Autodesk Fusion 360 part; units mm, degrees
note: some values were not read from the file. Set by a fixed rule: which sketch regions a step uses.
(part 3 of 20)
  spline S12 degree 5 poles (15.9204, -26.5997) (15.9199, -26.597) (15.9189, -26.5917) (15.9174, -26.5837) (15.9154, -26.5731) (15.913, -26.5599) (15.9105, -26.5467) (15.908, -26.5335) (15.9055, -26.5204) (15.9029, -26.5073) (15.9004, -26.4943) (15.8979, -26.4812) (15.8953, -26.4682) (15.8927, -26.4553) (15.8902, -26.4424) (15.8876, -26.4295) (15.885, -26.4166) (15.8824, -26.4038) (15.8798, -26.391) (15.8771, -26.3783) (15.8745, -26.3656) (15.8719, -26.3529) (15.8692, -26.3403) (15.8666, -26.3276) (15.8639, -26.3151) (15.8612, -26.3025) (15.8585, -26.29) (15.8558, -26.2776) (15.8531, -26.2651) (15.8504, -26.2528) (15.8477, -26.2404) (15.8449, -26.2281) (15.8422, -26.2158) (15.8394, -26.2035) (15.8367, -26.1913) (15.8339, -26.1792) (15.8311, -26.167) (15.8283, -26.1549) (15.8255, -26.1428) (15.8227, -26.1308) (15.8199, -26.1188) (15.8171, -26.1069) (15.8143, -26.095) (15.8115, -26.0831) (15.8086, -26.0712) (15.8058, -26.0594) (15.8029, -26.0477) (15.8001, -26.0359) (15.7972, -26.0242) (15.7943, -26.0126) (15.7914, -26.001) (15.7886, -25.9894) (15.7857, -25.9778) (15.7828, -25.9663) (15.7798, -25.9549) (15.7769, -25.9435) (15.774, -25.9321) (15.7711, -25.9207) (15.7682, -25.9094) (15.7652, -25.8982) (15.7623, -25.8869) (15.7593, -25.8757) (15.7564, -25.8646) (15.7534, -25.8535) (15.7504, -25.8424) (15.7475, -25.8314) (15.7445, -25.8204) (15.7415, -25.8094) (15.7385, -25.7985) (15.7355, -25.7877) (15.7325, -25.7768) (15.7295, -25.766) (15.7265, -25.7553) (15.7235, -25.7446) (15.7205, -25.7339) (15.7175, -25.7233) (15.7145, -25.7127) (15.7114, -25.7022) (15.7084, -25.6917) (15.7054, -25.6812) (15.7023, -25.6708) (15.6993, -25.6604) (15.6963, -25.6501) (15.6932, -25.6398) (15.6902, -25.6296) (15.6871, -25.6194) (15.6841, -25.6092) (15.681, -25.5991) (15.6779, -25.589) (15.6749, -25.579) (15.6718, -25.569) (15.6688, -25.559) (15.6657, -25.5491) (15.6626, -25.5393) (15.6596, -25.5294) (15.6565, -25.5197) (15.6534, -25.5099) (15.6503, -25.5003) (15.6473, -25.4906) (15.6442, -25.481) (15.6411, -25.4715) (15.638, -25.462) (15.635, -25.4525) (15.6319, -25.4431) (15.6288, -25.4337) (15.6257, -25.4244) (15.6227, -25.4151) (15.6196, -25.4059) (15.6165, -25.3967) (15.6134, -25.3876) (15.6104, -25.3785) (15.6073, -25.3694) (15.6042, -25.3604) (15.6012, -25.3515) (15.5981, -25.3426) (15.595, -25.3337) (15.592, -25.3249) (15.5889, -25.3161) (15.5859, -25.3074) (15.5828, -25.2988) (15.5798, -25.2901) (15.5767, -25.2816) (15.5737, -25.2731) (15.5706, -25.2646) (15.5676, -25.2562) (15.5645, -25.2478) (15.5615, -25.2394) (15.5585, -25.2312) (15.5555, -25.2229) (15.5524, -25.2148) (15.5494, -25.2066) (15.5464, -25.1986) (15.5434, -25.1905) (15.5404, -25.1826) (15.5374, -25.1746) (15.5344, -25.1668) (15.5315, -25.1589) (15.5285, -25.1512) (15.5255, -25.1434) (15.5226, -25.1358) (15.5196, -25.1282) (15.5166, -25.1206) (15.5137, -25.1131) (15.5108, -25.1056) (15.5078, -25.0982) (15.5049, -25.0909) (15.502, -25.0836) (15.4991, -25.0763) (15.4962, -25.0691) (15.4933, -25.062) (15.4905, -25.0549) (15.4876, -25.0479) (15.4848, -25.0409) (15.4819, -25.034) (15.4791, -25.0271) (15.4762, -25.0203) (15.4734, -25.0136) (15.4706, -25.0069) (15.4678, -25.0002) (15.4651, -24.9936) (15.4623, -24.9871) (15.4595, -24.9806) (15.4568, -24.9742) (15.4541, -24.9679) (15.4514, -24.9616) (15.4486, -24.9553) (15.446, -24.9492) (15.4433, -24.943) (15.4406, -24.937) (15.438, -24.931) (15.4353, -24.925) (15.4327, -24.9192) (15.4301, -24.9133) (15.4275, -24.9076) (15.425, -24.9019) (15.4224, -24.8962) (15.4199, -24.8907) (15.4174, -24.8852) (15.4149, -24.8797) (15.4124, -24.8743) (15.4099, -24.869) (15.4075, -24.8637) (15.405, -24.8585) (15.4026, -24.8534) (15.4002, -24.8483) (15.3979, -24.8433) (15.3955, -24.8384) (15.3932, -24.8335) (15.3909, -24.8287) (15.3886, -24.8239) (15.3863, -24.8193) (15.3841, -24.8147) (15.3819, -24.8101) (15.3797, -24.8056) (15.3775, -24.8012) (15.3754, -24.7969) (15.3733, -24.7926) (15.3712, -24.7884) (15.3691, -24.7843) (15.3671, -24.7802) (15.3651, -24.7763) (15.3631, -24.7723) (15.3611, -24.7685) (15.3592, -24.7647) (15.3573, -24.761) (15.3554, -24.7574) (15.3536, -24.7539) (15.3518, -24.7504) (15.35, -24.747) (15.3482, -24.7437) (15.3465, -24.7404) (15.3449, -24.7372) (15.3432, -24.7341) (15.3416, -24.7311) (15.34, -24.7282) (15.3385, -24.7253) (15.337, -24.7225) (15.3355, -24.7198) (15.3341, -24.7172) (15.3327, -24.7147) (15.3313, -24.7122) (15.33, -24.7099) (15.3287, -24.7076) (15.3275, -24.7054) (15.3263, -24.7033) (15.3252, -24.7012) (15.3241, -24.6993) (15.323, -24.6974) (15.322, -24.6956) (15.321, -24.694) (15.3201, -24.6924) (15.3193, -24.6909) (15.3184, -24.6895) (15.3177, -24.6881) (15.3169, -24.6869) (15.3163, -24.6858) (15.3157, -24.6848) (15.3151, -24.6838) (15.3146, -24.683) (15.3142, -24.6822) (15.3138, -24.6816) (15.3135, -24.6812) (15.3133, -24.6809) (15.3132, -24.6807) (15.3132, -24.6806) knots -1 -1 -1 -1 -1 -1 -0.99583333 -0.99166667 -0.9875 -0.98333333 -0.97916667 -0.975 -0.97083333 -0.96666667 -0.9625 -0.95833333 -0.95416667 -0.95 -0.94583333 -0.94166667 -0.9375 -0.93333333 -0.92916667 -0.925 -0.92083333 -0.91666667 -0.9125 -0.90833333 -0.90416667 -0.9 -0.89583333 -0.89166667 -0.8875 -0.88333333 -0.87916667 -0.875 -0.87083333 -0.86666667 -0.8625 -0.85833333 -0.85416667 -0.85 -0.84583333 -0.84166667 -0.8375 -0.83333333 -0.82916667 -0.825 -0.82083333 -0.81666667 -0.8125 -0.80833333 -0.80416667 -0.8 -0.79583333 -0.79166667 -0.7875 -0.78333333 -0.77916667 -0.775 -0.77083333 -0.76666667 -0.7625 -0.75833333 -0.75416667 -0.75 -0.74583333 -0.74166667 -0.7375 -0.73333333 -0.72916667 -0.725 -0.72083333 -0.71666667 -0.7125 -0.70833333 -0.70416667 -0.7 -0.69583333 -0.69166667 -0.6875 -0.68333333 -0.67916667 -0.675 -0.67083333 -0.66666667 -0.6625 -0.65833333 -0.65416667 -0.65 -0.64583333 -0.64166667 -0.6375 -0.63333333 -0.62916667 -0.625 -0.62083333 -0.61666667 -0.6125 -0.60833333 -0.60416667 -0.6 -0.59583333 -0.59166667 -0.5875 -0.58333333 -0.57916667 -0.575 -0.57083333 -0.56666667 -0.5625 -0.55833333 -0.55416667 -0.55 -0.54583333 -0.54166667 -0.5375 -0.53333333 -0.52916667 -0.525 -0.52083333 -0.51666667 -0.5125 -0.50833333 -0.50416667 -0.5 -0.49583333 -0.49166667 -0.4875 -0.48333333 -0.47916667 -0.475 -0.47083333 -0.46666667 -0.4625 -0.45833333 -0.45416667 -0.45 -0.44583333 -0.44166667 -0.4375 -0.43333333 -0.42916667 -0.425 -0.42083333 -0.41666667 -0.4125 -0.40833333 -0.40416667 -0.4 -0.39583333 -0.39166667 -0.3875 -0.38333333 -0.37916667 -0.375 -0.37083333 -0.36666667 -0.3625 -0.35833333 -0.35416667 -0.35 -0.34583333 -0.34166667 -0.3375 -0.33333333 -0.32916667 -0.325 -0.32083333 -0.31666667 -0.3125 -0.30833333 -0.30416667 -0.3 -0.29583333 -0.29166667 -0.2875 -0.28333333 -0.27916667 -0.275 -0.27083333 -0.26666667 -0.2625 -0.25833333 -0.25416667 -0.25 -0.24583333 -0.24166667 -0.2375 -0.23333333 -0.22916667 -0.225 -0.22083333 -0.21666667 -0.2125 -0.20833333 -0.20416667 -0.2 -0.19583333 -0.19166667 -0.1875 -0.18333333 -0.17916667 -0.175 -0.17083333 -0.16666667 -0.1625 -0.15833333 -0.15416667 -0.15 -0.14583333 -0.14166667 -0.1375 -0.13333333 -0.12916667 -0.125 -0.12083333 -0.11666667 -0.1125 -0.10833333 -0.10416667 -0.1 -0.09583333 -0.09166667 -0.0875 -0.08333333 -0.07916667 -0.075 -0.07083333 -0.06666667 -0.0625 -0.05833333 -0.05416667 -0.05 -0.04583333 -0.04166667 -0.0375 -0.03333333 -0.02916667 -0.025 -0.02083333 -0.01666667 -0.0125 -0.00833333 -0.00416667 0 0 0 0 0 0
  line L22 (18.7401, 22.1898) -> (18.5501, 21.9649)
  line L23 (9.8472, -27.3251) -> (9.8469, -27.3243)
  arc A11 (15.1575, -24.4297) -> (16.1526, -23.7836) centre (0, 0) ccw
  arc A12 (15.0758, -27.0873) -> (15.9204, -26.5997) centre (0, 0) ccw
  line L24 (16.318, -24.0271) -> (16.3184, -24.0278)
  line L25 (16.1526, -23.7836) -> (16.318, -24.0271)
  line L26 (17.8086, 22.9441) -> (17.8091, 22.9448)
  spline S13 degree 5 poles (24.0278, 16.3184) (24.0279, 16.3185) (24.0281, 16.3186) (24.0283, 16.3188) (24.0287, 16.3191) (24.0294, 16.3195) (24.0301, 16.32) (24.0309, 16.3206) (24.0317, 16.3212) (24.0327, 16.3219) (24.0338, 16.3227) (24.035, 16.3235) (24.0362, 16.3244) (24.0375, 16.3253) (24.0389, 16.3263) (24.0404, 16.3274) (24.042, 16.3286) (24.0436, 16.3298) (24.0453, 16.331) (24.0471, 16.3324) (24.049, 16.3338) (24.051, 16.3352) (24.053, 16.3367) (24.0551, 16.3383) (24.0572, 16.3399) (24.0595, 16.3416) (24.0618, 16.3434) (24.0641, 16.3452) (24.0666, 16.3471) (24.0691, 16.349) (24.0717, 16.351) (24.0743, 16.353) (24.077, 16.3551) (24.0798, 16.3573) (24.0826, 16.3595) (24.0855, 16.3618) (24.0884, 16.3641) (24.0914, 16.3665) (24.0945, 16.3689) (24.0976, 16.3714) (24.1008, 16.374) (24.104, 16.3766) (24.1073, 16.3792) (24.1107, 16.3819) (24.1141, 16.3847) (24.1176, 16.3875) (24.1211, 16.3904) (24.1246, 16.3933) (24.1283, 16.3963) (24.1319, 16.3994) (24.1356, 16.4024) (24.1394, 16.4056) (24.1432, 16.4088) (24.1471, 16.412) (24.151, 16.4153) (24.155, 16.4187) (24.159, 16.4221) (24.1631, 16.4256) (24.1672, 16.4291) (24.1713, 16.4326) (24.1755, 16.4362) (24.1798, 16.4399) (24.1841, 16.4436) (24.1884, 16.4474) (24.1928, 16.4512) (24.1972, 16.455) (24.2017, 16.459) (24.2062, 16.4629) (24.2107, 16.4669) (24.2153, 16.471) (24.2199, 16.4751) (24.2246, 16.4793) (24.2293, 16.4835) (24.234, 16.4877) (24.2388, 16.492) (24.2436, 16.4964) (24.2485, 16.5008) (24.2534, 16.5053) (24.2583, 16.5098) (24.2633, 16.5143) (24.2683, 16.5189) (24.2733, 16.5236) (24.2784, 16.5282) (24.2835, 16.533) (24.2887, 16.5378) (24.2939, 16.5426) (24.2991, 16.5475) (24.3043, 16.5524) (24.3096, 16.5574) (24.3149, 16.5624) (24.3203, 16.5675) (24.3257, 16.5726) (24.3311, 16.5778) (24.3365, 16.583) (24.342, 16.5882) (24.3475, 16.5935) (24.353, 16.5989) (24.3586, 16.6043) (24.3642, 16.6097) (24.3698, 16.6152) (24.3755, 16.6207) (24.3812, 16.6263) (24.3869, 16.6319) (24.3926, 16.6376) (24.3984, 16.6433) (24.4042, 16.6491) (24.41, 16.6549) (24.4159, 16.6607) (24.4218, 16.6666) (24.4277, 16.6725) (24.4336, 16.6785) (24.4395, 16.6845) (24.4455, 16.6906) (24.4515, 16.6967) (24.4576, 16.7029) (24.4636, 16.7091) (24.4697, 16.7153) (24.4758, 16.7216) (24.482, 16.7279) (24.4881, 16.7343) (24.4943, 16.7407) (24.5005, 16.7472) (24.5067, 16.7537) (24.513, 16.7602) (24.5192, 16.7668) (24.5255, 16.7735) (24.5319, 16.7801) (24.5382, 16.7869) (24.5446, 16.7936) (24.5509, 16.8004) (24.5573, 16.8073) (24.5638, 16.8142) (24.5702, 16.8211) (24.5767, 16.8281) (24.5831, 16.8351) (24.5897, 16.8421) (24.5962, 16.8492) (24.6027, 16.8564) (24.6093, 16.8636) (24.6159, 16.8708) (24.6225, 16.8781) (24.6291, 16.8854) (24.6357, 16.8927) (24.6424, 16.9001) (24.6491, 16.9075) (24.6558, 16.915) (24.6625, 16.9225) (24.6692, 16.9301) (24.6759, 16.9377) (24.6827, 16.9453) (24.6895, 16.953) (24.6963, 16.9607) (24.7031, 16.9685) (24.7099, 16.9763) (24.7168, 16.9841) (24.7236, 16.992) (24.7305, 16.9999) (24.7374, 17.0079) (24.7443, 17.0159) (24.7512, 17.0239) (24.7582, 17.032) (24.7651, 17.0401) (24.7721, 17.0483) (24.7791, 17.0565) (24.7861, 17.0647) (24.7931, 17.073) (24.8001, 17.0813) (24.8071, 17.0897) (24.8142, 17.0981) (24.8212, 17.1065) (24.8283, 17.115) (24.8354, 17.1235) (24.8425, 17.1321) (24.8496, 17.1407) (24.8568, 17.1493) (24.8639, 17.158) (24.8711, 17.1667) (24.8782, 17.1754) (24.8854, 17.1842) (24.8926, 17.1931) (24.8998, 17.2019) (24.907, 17.2108) (24.9142, 17.2198) (24.9215, 17.2288) (24.9287, 17.2378) (24.936, 17.2469) (24.9432, 17.2559) (24.9505, 17.2651) (24.9578, 17.2743) (24.9651, 17.2835) (24.9724, 17.2927) (24.9797, 17.302) (24.9871, 17.3113) (24.9944, 17.3207) (25.0017, 17.3301) (25.0091, 17.3395) (25.0165, 17.349) (25.0238, 17.3585) (25.0312, 17.3681) (25.0386, 17.3777) (25.046, 17.3873) (25.0534, 17.397) (25.0609, 17.4067) (25.0683, 17.4164) (25.0757, 17.4262) (25.0832, 17.436) (25.0906, 17.4458) (25.0981, 17.4557) (25.1055, 17.4657) (25.113, 17.4756) (25.1205, 17.4856) (25.128, 17.4956) (25.1355, 17.5057) (25.143, 17.5158) (25.1505, 17.526) (25.158, 17.5361) (25.1655, 17.5464) (25.1731, 17.5566) (25.1806, 17.5669) (25.1881, 17.5772) (25.1957, 17.5876) (25.2032, 17.598) (25.2108, 17.6084) (25.2184, 17.6189) (25.2259, 17.6294) (25.2335, 17.6399) (25.2411, 17.6505) (25.2487, 17.6611) (25.2563, 17.6718) (25.2639, 17.6825) (25.2715, 17.6932) (25.2791, 17.7039) (25.2867, 17.7147) (25.2943, 17.7256) (25.3019, 17.7364) (25.3096, 17.7473) (25.3172, 17.7583) (25.3248, 17.7692) (25.3325, 17.7802) (25.3401, 17.7913) (25.3477, 17.8023) (25.3539, 17.8112) (25.3584, 17.8179) (25.3615, 17.8224) (25.363, 17.8246) knots 0 0 0 0 0 0 0.00416667 0.00833333 0.0125 0.01666667 0.02083333 0.025 0.02916667 0.03333333 0.0375 0.04166667 0.04583333 0.05 0.05416667 0.05833333 0.0625 0.06666667 0.07083333 0.075 0.07916667 0.08333333 0.0875 0.09166667 0.09583333 0.1 0.10416667 0.10833333 0.1125 0.11666667 0.12083333 0.125 0.12916667 0.13333333 0.1375 0.14166667 0.14583333 0.15 0.15416667 0.15833333 0.1625 0.16666667 0.17083333 0.175 0.17916667 0.18333333 0.1875 0.19166667 0.19583333 0.2 0.20416667 0.20833333 0.2125 0.21666667 0.22083333 0.225 0.22916667 0.23333333 0.2375 0.24166667 0.24583333 0.25 0.25416667 0.25833333 0.2625 0.26666667 0.27083333 0.275 0.27916667 0.28333333 0.2875 0.29166667 0.29583333 0.3 0.30416667 0.30833333 0.3125 0.31666667 0.32083333 0.325 0.32916667 0.33333333 0.3375 0.34166667 0.34583333 0.35 0.35416667 0.35833333 0.3625 0.36666667 0.37083333 0.375 0.37916667 0.38333333 0.3875 0.39166667 0.39583333 0.4 0.40416667 0.40833333 0.4125 0.41666667 0.42083333 0.425 0.42916667 0.43333333 0.4375 0.44166667 0.44583333 0.45 0.45416667 0.45833333 0.4625 0.46666667 0.47083333 0.475 0.47916667 0.48333333 0.4875 0.49166667 0.49583333 0.5 0.50416667 0.50833333 0.5125 0.51666667 0.52083333 0.525 0.52916667 0.53333333 0.5375 0.54166667 0.54583333 0.55 0.55416667 0.55833333 0.5625 0.56666667 0.57083333 0.575 0.57916667 0.58333333 0.5875 0.59166667 0.59583333 0.6 0.60416667 0.60833333 0.6125 0.61666667 0.62083333 0.625 0.62916667 0.63333333 0.6375 0.64166667 0.64583333 0.65 0.65416667 0.65833333 0.6625 0.66666667 0.67083333 0.675 0.67916667 0.68333333 0.6875 0.69166667 0.69583333 0.7 0.70416667 0.70833333 0.7125 0.71666667 0.72083333 0.725 0.72916667 0.73333333 0.7375 0.74166667 0.74583333 0.75 0.75416667 0.75833333 0.7625 0.76666667 0.77083333 0.775 0.77916667 0.78333333 0.7875 0.79166667 0.79583333 0.8 0.80416667 0.80833333 0.8125 0.81666667 0.82083333 0.825 0.82916667 0.83333333 0.8375 0.84166667 0.84583333 0.85 0.85416667 0.85833333 0.8625 0.86666667 0.87083333 0.875 0.87916667 0.88333333 0.8875 0.89166667 0.89583333 0.9 0.90416667 0.90833333 0.9125 0.91666667 0.92083333 0.925 0.92916667 0.93333333 0.9375 0.94166667 0.94583333 0.95 0.95416667 0.95833333 0.9625 0.96666667 0.97083333 0.975 0.97916667 0.98333333 0.9875 0.99166667 0.99583333 1 1 1 1 1 1
  line L27 (15.3128, -24.6799) -> (15.1575, -24.4297)
  spline S14 degree 5 poles (13.7175, -25.6019) (13.7175, -25.602) (13.7176, -25.6022) (13.7178, -25.6025) (13.718, -25.6029) (13.7184, -25.6036) (13.7188, -25.6043) (13.7193, -25.6052) (13.7198, -25.6061) (13.7204, -25.6072) (13.721, -25.6083) (13.7217, -25.6096) (13.7225, -25.6109) (13.7233, -25.6123) (13.7242, -25.6138) (13.7251, -25.6154) (13.7261, -25.6171) (13.7271, -25.6188) (13.7282, -25.6207) (13.7293, -25.6226) (13.7305, -25.6246) (13.7317, -25.6267) (13.733, -25.6289) (13.7344, -25.6311) (13.7358, -25.6334) (13.7372, -25.6358) (13.7387, -25.6383) (13.7403, -25.6409) (13.7419, -25.6435) (13.7435, -25.6462) (13.7452, -25.6489) (13.747, -25.6518) (13.7488, -25.6547) (13.7506, -25.6577) (13.7526, -25.6607) (13.7545, -25.6638) (13.7565, -25.667) (13.7586, -25.6702) (13.7607, -25.6735) (13.7628, -25.6769) (13.765, -25.6803) (13.7673, -25.6838) (13.7696, -25.6874) (13.7719, -25.691) (13.7743, -25.6947) (13.7768, -25.6984) (13.7793, -25.7022) (13.7818, -25.706) (13.7844, -25.71) (13.787, -25.7139) (13.7897, -25.718) (13.7925, -25.722) (13.7952, -25.7262) (13.7981, -25.7304) (13.8009, -25.7346) (13.8039, -25.7389) (13.8068, -25.7432) (13.8098, -25.7476) (13.8129, -25.7521) (13.816, -25.7566) (13.8192, -25.7612) (13.8224, -25.7658) (13.8256, -25.7704) (13.8289, -25.7751) (13.8322, -25.7799) (13.8356, -25.7847) (13.839, -25.7895) (13.8425, -25.7944) (13.846, -25.7993) (13.8496, -25.8043) (13.8532, -25.8093) (13.8568, -25.8144) (13.8605, -25.8195) (13.8643, -25.8247) (13.8681, -25.8299) (13.8719, -25.8352) (13.8758, -25.8405) (13.8797, -25.8458) (13.8836, -25.8512) (13.8876, -25.8566) (13.8917, -25.8621) (13.8958, -25.8676) (13.8999, -25.8731) (13.9041, -25.8787) (13.9083, -25.8843) (13.9126, -25.89) (13.9169, -25.8957) (13.9213, -25.9014) (13.9257, -25.9072) (13.9301, -25.913) (13.9346, -25.9188) (13.9391, -25.9247) (13.9437, -25.9306) (13.9483, -25.9366) (13.9529, -25.9426) (13.9576, -25.9486) (13.9624, -25.9547) (13.9672, -25.9608) (13.972, -25.9669) (13.9769, -25.9731) (13.9818, -25.9793) (13.9867, -25.9855) (13.9917, -25.9918) (13.9967, -25.9981) (14.0018, -26.0044) (14.0069, -26.0108) (14.0121, -26.0172) (14.0173, -26.0236) (14.0225, -26.0301) (14.0278, -26.0366) (14.0332, -26.0431) (14.0385, -26.0497) (14.0439, -26.0563) (14.0494, -26.0629) (14.0549, -26.0695) (14.0604, -26.0762) (14.066, -26.0829) (14.0716, -26.0896) (14.0772, -26.0964) (14.0829, -26.1032) (14.0887, -26.11) (14.0945, -26.1168) (14.1003, -26.1237) (14.1061, -26.1306) (14.112, -26.1375) (14.118, -26.1445) (14.1239, -26.1515) (14.13, -26.1585) (14.136, -26.1655) (14.1421, -26.1726) (14.1483, -26.1796) (14.1544, -26.1868) (14.1607, -26.1939) (14.1669, -26.201) (14.1732, -26.2082) (14.1796, -26.2154) (14.1859, -26.2227) (14.1924, -26.2299) (14.1988, -26.2372) (14.2053, -26.2445) (14.2119, -26.2518) (14.2184, -26.2592) (14.225, -26.2665) (14.2317, -26.2739) (14.2384, -26.2813) (14.2451, -26.2888) (14.2519, -26.2962) (14.2587, -26.3037) (14.2656, -26.3112) (14.2724, -26.3188) (14.2794, -26.3263) (14.2863, -26.3339) (14.2933, -26.3414) (14.3004, -26.3491) (14.3075, -26.3567) (14.3146, -26.3643) (14.3217, -26.372) (14.3289, -26.3797) (14.3362, -26.3874) (14.3435, -26.3951) (14.3508, -26.4029) (14.3581, -26.4106) (14.3655, -26.4184) (14.3729, -26.4262) (14.3804, -26.434) (14.3879, -26.4419) (14.3954, -26.4497) (14.403, -26.4576) (14.4106, -26.4655) (14.4183, -26.4734) (14.426, -26.4813) (14.4337, -26.4893) (14.4415, -26.4972) (14.4493, -26.5052) (14.4571, -26.5132) (14.465, -26.5212) (14.4729, -26.5292) (14.4809, -26.5373) (14.4889, -26.5453) (14.4969, -26.5534) (14.505, -26.5615) (14.5131, -26.5696) (14.5212, -26.5777) (14.5294, -26.5858) (14.5376, -26.594) (14.5459, -26.6022) (14.5541, -26.6103) (14.5625, -26.6185) (14.5708, -26.6267) (14.5792, -26.635) (14.5877, -26.6432) (14.5961, -26.6514) (14.6046, -26.6597) (14.6132, -26.668) (14.6218, -26.6763) (14.6304, -26.6846) (14.639, -26.6929) (14.6477, -26.7012) (14.6565, -26.7096) (14.6652, -26.7179) (14.674, -26.7263) (14.6829, -26.7347) (14.6917, -26.7431) (14.7006, -26.7515) (14.7096, -26.7599) (14.7186, -26.7683) (14.7276, -26.7767) (14.7366, -26.7852) (14.7457, -26.7937) (14.7549, -26.8021) (14.764, -26.8106) (14.7732, -26.8191) (14.7824, -26.8276) (14.7917, -26.8361) (14.801, -26.8447) (14.8104, -26.8532) (14.8197, -26.8618) (14.8291, -26.8703) (14.8386, -26.8789) (14.8481, -26.8875) (14.8576, -26.8961) (14.8671, -26.9047) (14.8767, -26.9133) (14.8863, -26.9219) (14.896, -26.9305) (14.9057, -26.9392) (14.9154, -26.9478) (14.9252, -26.9565) (14.935, -26.9651) (14.9448, -26.9738) (14.9547, -26.9825) (14.9646, -26.9912) (14.9745, -26.9999) (14.9845, -27.0086) (14.9945, -27.0173) (15.0045, -27.026) (15.0146, -27.0347) (15.0247, -27.0435) (15.0349, -27.0522) (15.045, -27.061) (15.0553, -27.0697) (15.0635, -27.0767) (15.0696, -27.082) (15.0737, -27.0855) (15.0758, -27.0873) knots 0 0 0 0 0 0 0.00416667 0.00833333 0.0125 0.01666667 0.02083333 0.025 0.02916667 0.03333333 0.0375 0.04166667 0.04583333 0.05 0.05416667 0.05833333 0.0625 0.06666667 0.07083333 0.075 0.07916667 0.08333333 0.0875 0.09166667 0.09583333 0.1 0.10416667 0.10833333 0.1125 0.11666667 0.12083333 0.125 0.12916667 0.13333333 0.1375 0.14166667 0.14583333 0.15 0.15416667 0.15833333 0.1625 0.16666667 0.17083333 0.175 0.17916667 0.18333333 0.1875 0.19166667 0.19583333 0.2 0.20416667 0.20833333 0.2125 0.21666667 0.22083333 0.225 0.22916667 0.23333333 0.2375 0.24166667 0.24583333 0.25 0.25416667 0.25833333 0.2625 0.26666667 0.27083333 0.275 0.27916667 0.28333333 0.2875 0.29166667 0.29583333 0.3 0.30416667 0.30833333 0.3125 0.31666667 0.32083333 0.325 0.32916667 0.33333333 0.3375 0.34166667 0.34583333 0.35 0.35416667 0.35833333 0.3625 0.36666667 0.37083333 0.375 0.37916667 0.38333333 0.3875 0.39166667 0.39583333 0.4 0.40416667 0.40833333 0.4125 0.41666667 0.42083333 0.425 0.42916667 0.43333333 0.4375 0.44166667 0.44583333 0.45 0.45416667 0.45833333 0.4625 0.46666667 0.47083333 0.475 0.47916667 0.48333333 0.4875 0.49166667 0.49583333 0.5 0.50416667 0.50833333 0.5125 0.51666667 0.52083333 0.525 0.52916667 0.53333333 0.5375 0.54166667 0.54583333 0.55 0.55416667 0.55833333 0.5625 0.56666667 0.57083333 0.575 0.57916667 0.58333333 0.5875 0.59166667 0.59583333 0.6 0.60416667 0.60833333 0.6125 0.61666667 0.62083333 0.625 0.62916667 0.63333333 0.6375 0.64166667 0.64583333 0.65 0.65416667 0.65833333 0.6625 0.66666667 0.67083333 0.675 0.67916667 0.68333333 0.6875 0.69166667 0.69583333 0.7 0.70416667 0.70833333 0.7125 0.71666667 0.72083333 0.725 0.72916667 0.73333333 0.7375 0.74166667 0.74583333 0.75 0.75416667 0.75833333 0.7625 0.76666667 0.77083333 0.775 0.77916667 0.78333333 0.7875 0.79166667 0.79583333 0.8 0.80416667 0.80833333 0.8125 0.81666667 0.82083333 0.825 0.82916667 0.83333333 0.8375 0.84166667 0.84583333 0.85 0.85416667 0.85833333 0.8625 0.86666667 0.87083333 0.875 0.87916667 0.88333333 0.8875 0.89166667 0.89583333 0.9 0.90416667 0.90833333 0.9125 0.91666667 0.92083333 0.925 0.92916667 0.93333333 0.9375 0.94166667 0.94583333 0.95 0.95416667 0.95833333 0.9625 0.96666667 0.97083333 0.975 0.97916667 0.98333333 0.9875 0.99166667 0.99583333 1 1 1 1 1 1
  line L28 (15.3132, -24.6806) -> (15.3128, -24.6799)
  spline S15 degree 5 poles (16.3184, -24.0278) (16.3185, -24.0279) (16.3186, -24.0281) (16.3188, -24.0283) (16.3191, -24.0287) (16.3195, -24.0294) (16.32, -24.0301) (16.3206, -24.0309) (16.3212, -24.0317) (16.3219, -24.0327) (16.3227, -24.0338) (16.3235, -24.035) (16.3244, -24.0362) (16.3253, -24.0375) (16.3263, -24.0389) (16.3274, -24.0404) (16.3286, -24.042) (16.3298, -24.0436) (16.331, -24.0453) (16.3324, -24.0471) (16.3338, -24.049) (16.3352, -24.051) (16.3367, -24.053) (16.3383, -24.0551) (16.3399, -24.0572) (16.3416, -24.0595) (16.3434, -24.0618) (16.3452, -24.0641) (16.3471, -24.0666) (16.349, -24.0691) (16.351, -24.0717) (16.353, -24.0743) (16.3551, -24.077) (16.3573, -24.0798) (16.3595, -24.0826) (16.3618, -24.0855) (16.3641, -24.0884) (16.3665, -24.0914) (16.3689, -24.0945) (16.3714, -24.0976) (16.374, -24.1008) (16.3766, -24.104) (16.3792, -24.1073) (16.3819, -24.1107) (16.3847, -24.1141) (16.3875, -24.1176) (16.3904, -24.1211) (16.3933, -24.1246) (16.3963, -24.1283) (16.3994, -24.1319) (16.4024, -24.1356) (16.4056, -24.1394) (16.4088, -24.1432) (16.412, -24.1471) (16.4153, -24.151) (16.4187, -24.155) (16.4221, -24.159) (16.4256, -24.1631) (16.4291, -24.1672) (16.4326, -24.1713) (16.4362, -24.1755) (16.4399, -24.1798) (16.4436, -24.1841) (16.4474, -24.1884) (16.4512, -24.1928) (16.455, -24.1972) (16.459, -24.2017) (16.4629, -24.2062) (16.4669, -24.2107) (16.471, -24.2153) (16.4751, -24.2199) (16.4793, -24.2246) (16.4835, -24.2293) (16.4877, -24.234) (16.492, -24.2388) (16.4964, -24.2436) (16.5008, -24.2485) (16.5053, -24.2534) (16.5098, -24.2583) (16.5143, -24.2633) (16.5189, -24.2683) (16.5236, -24.2733) (16.5282, -24.2784) (16.533, -24.2835) (16.5378, -24.2887) (16.5426, -24.2939) (16.5475, -24.2991) (16.5524, -24.3043) (16.5574, -24.3096) (16.5624, -24.3149) (16.5675, -24.3203) (16.5726, -24.3257) (16.5778, -24.3311) (16.583, -24.3365) (16.5882, -24.342) (16.5935, -24.3475) (16.5989, -24.353) (16.6043, -24.3586) (16.6097, -24.3642) (16.6152, -24.3698) (16.6207, -24.3755) (16.6263, -24.3812) (16.6319, -24.3869) (16.6376, -24.3926) (16.6433, -24.3984) (16.6491, -24.4042) (16.6549, -24.41) (16.6607, -24.4159) (16.6666, -24.4218) (16.6725, -24.4277) (16.6785, -24.4336) (16.6845, -24.4395) (16.6906, -24.4455) (16.6967, -24.4515) (16.7029, -24.4576) (16.7091, -24.4636) (16.7153, -24.4697) (16.7216, -24.4758) (16.7279, -24.482) (16.7343, -24.4881) (16.7407, -24.4943) (16.7472, -24.5005) (16.7537, -24.5067) (16.7602, -24.513) (16.7668, -24.5192) (16.7735, -24.5255) (16.7801, -24.5319) (16.7869, -24.5382) (16.7936, -24.5446) (16.8004, -24.5509) (16.8073, -24.5573) (16.8142, -24.5638) (16.8211, -24.5702) (16.8281, -24.5767) (16.8351, -24.5831) (16.8421, -24.5897) (16.8492, -24.5962) (16.8564, -24.6027) (16.8636, -24.6093) (16.8708, -24.6159) (16.8781, -24.6225) (16.8854, -24.6291) (16.8927, -24.6357) (16.9001, -24.6424) (16.9075, -24.6491) (16.915, -24.6558) (16.9225, -24.6625) (16.9301, -24.6692) (16.9377, -24.6759) (16.9453, -24.6827) (16.953, -24.6895) (16.9607, -24.6963) (16.9685, -24.7031) (16.9763, -24.7099) (16.9841, -24.7168) (16.992, -24.7236) (16.9999, -24.7305) (17.0079, -24.7374) (17.0159, -24.7443) (17.0239, -24.7512) (17.032, -24.7582) (17.0401, -24.7651) (17.0483, -24.7721) (17.0565, -24.7791) (17.0647, -24.7861) (17.073, -24.7931) (17.0813, -24.8001) (17.0897, -24.8071) (17.0981, -24.8142) (17.1065, -24.8212) (17.115, -24.8283) (17.1235, -24.8354) (17.1321, -24.8425) (17.1407, -24.8496) (17.1493, -24.8568) (17.158, -24.8639) (17.1667, -24.8711) (17.1754, -24.8782) (17.1842, -24.8854) (17.1931, -24.8926) (17.2019, -24.8998) (17.2108, -24.907) (17.2198, -24.9142) (17.2288, -24.9215) (17.2378, -24.9287) (17.2469, -24.936) (17.2559, -24.9432) (17.2651, -24.9505) (17.2743, -24.9578) (17.2835, -24.9651) (17.2927, -24.9724) (17.302, -24.9797) (17.3113, -24.9871) (17.3207, -24.9944) (17.3301, -25.0017) (17.3395, -25.0091) (17.349, -25.0165) (17.3585, -25.0238) (17.3681, -25.0312) (17.3777, -25.0386) (17.3873, -25.046) (17.397, -25.0534) (17.4067, -25.0609) (17.4164, -25.0683) (17.4262, -25.0757) (17.436, -25.0832) (17.4458, -25.0906) (17.4557, -25.0981) (17.4657, -25.1055) (17.4756, -25.113) (17.4856, -25.1205) (17.4956, -25.128) (17.5057, -25.1355) (17.5158, -25.143) (17.526, -25.1505) (17.5361, -25.158) (17.5464, -25.1655) (17.5566, -25.1731) (17.5669, -25.1806) (17.5772, -25.1881) (17.5876, -25.1957) (17.598, -25.2032) (17.6084, -25.2108) (17.6189, -25.2184) (17.6294, -25.2259) (17.6399, -25.2335) (17.6505, -25.2411) (17.6611, -25.2487) (17.6718, -25.2563) (17.6825, -25.2639) (17.6932, -25.2715) (17.7039, -25.2791) (17.7147, -25.2867) (17.7256, -25.2943) (17.7364, -25.3019) (17.7473, -25.3096) (17.7583, -25.3172) (17.7692, -25.3248) (17.7802, -25.3325) (17.7913, -25.3401) (17.8023, -25.3477) (17.8112, -25.3539) (17.8179, -25.3584) (17.8224, -25.3615) (17.8246, -25.363) knots 0 0 0 0 0 0 0.00416667 0.00833333 0.0125 0.01666667 0.02083333 0.025 0.02916667 0.03333333 0.0375 0.04166667 0.04583333 0.05 0.05416667 0.05833333 0.0625 0.06666667 0.07083333 0.075 0.07916667 0.08333333 0.0875 0.09166667 0.09583333 0.1 0.10416667 0.10833333 0.1125 0.11666667 0.12083333 0.125 0.12916667 0.13333333 0.1375 0.14166667 0.14583333 0.15 0.15416667 0.15833333 0.1625 0.16666667 0.17083333 0.175 0.17916667 0.18333333 0.1875 0.19166667 0.19583333 0.2 0.20416667 0.20833333 0.2125 0.21666667 0.22083333 0.225 0.22916667 0.23333333 0.2375 0.24166667 0.24583333 0.25 0.25416667 0.25833333 0.2625 0.26666667 0.27083333 0.275 0.27916667 0.28333333 0.2875 0.29166667 0.29583333 0.3 0.30416667 0.30833333 0.3125 0.31666667 0.32083333 0.325 0.32916667 0.33333333 0.3375 0.34166667 0.34583333 0.35 0.35416667 0.35833333 0.3625 0.36666667 0.37083333 0.375 0.37916667 0.38333333 0.3875 0.39166667 0.39583333 0.4 0.40416667 0.40833333 0.4125 0.41666667 0.42083333 0.425 0.42916667 0.43333333 0.4375 0.44166667 0.44583333 0.45 0.45416667 0.45833333 0.4625 0.46666667 0.47083333 0.475 0.47916667 0.48333333 0.4875 0.49166667 0.49583333 0.5 0.50416667 0.50833333 0.5125 0.51666667 0.52083333 0.525 0.52916667 0.53333333 0.5375 0.54166667 0.54583333 0.55 0.55416667 0.55833333 0.5625 0.56666667 0.57083333 0.575 0.57916667 0.58333333 0.5875 0.59166667 0.59583333 0.6 0.60416667 0.60833333 0.6125 0.61666667 0.62083333 0.625 0.62916667 0.63333333 0.6375 0.64166667 0.64583333 0.65 0.65416667 0.65833333 0.6625 0.66666667 0.67083333 0.675 0.67916667 0.68333333 0.6875 0.69166667 0.69583333 0.7 0.70416667 0.70833333 0.7125 0.71666667 0.72083333 0.725 0.72916667 0.73333333 0.7375 0.74166667 0.74583333 0.75 0.75416667 0.75833333 0.7625 0.76666667 0.77083333 0.775 0.77916667 0.78333333 0.7875 0.79166667 0.79583333 0.8 0.80416667 0.80833333 0.8125 0.81666667 0.82083333 0.825 0.82916667 0.83333333 0.8375 0.84166667 0.84583333 0.85 0.85416667 0.85833333 0.8625 0.86666667 0.87083333 0.875 0.87916667 0.88333333 0.8875 0.89166667 0.89583333 0.9 0.90416667 0.90833333 0.9125 0.91666667 0.92083333 0.925 0.92916667 0.93333333 0.9375 0.94166667 0.94583333 0.95 0.95416667 0.95833333 0.9625 0.96666667 0.97083333 0.975 0.97916667 0.98333333 0.9875 0.99166667 0.99583333 1 1 1 1 1 1
  line L29 (20.1094, 20.9569) -> (20.11, 20.9575)
  line L30 (20.9575, 20.11) -> (20.9569, 20.1094)
  line L31 (10.8547, -26.6221) -> (10.9659, -26.8948)
  line L32 (10.9659, -26.8948) -> (10.9662, -26.8955)
  arc A13 (-25.363, -17.8246) -> (-24.7898, -18.6136) centre (0, 0) ccw
  line L33 (-27.3243, -9.8469) -> (-27.0473, -9.7471)
  line L34 (-20.9575, -20.11) -> (-20.9569, -20.1094)
  line L35 (-26.8948, -10.9659) -> (-26.8955, -10.9662)
  spline S16 degree 5 poles (-24.0278, -16.3184) (-24.0279, -16.3185) (-24.0281, -16.3186) (-24.0283, -16.3188) (-24.0287, -16.3191) (-24.0294, -16.3195) (-24.0301, -16.32) (-24.0309, -16.3206) (-24.0317, -16.3212) (-24.0327, -16.3219) (-24.0338, -16.3227) (-24.035, -16.3235) (-24.0362, -16.3244) (-24.0375, -16.3253) (-24.0389, -16.3263) (-24.0404, -16.3274) (-24.042, -16.3286) (-24.0436, -16.3298) (-24.0453, -16.331) (-24.0471, -16.3324) (-24.049, -16.3338) (-24.051, -16.3352) (-24.053, -16.3367) (-24.0551, -16.3383) (-24.0572, -16.3399) (-24.0595, -16.3416) (-24.0618, -16.3434) (-24.0641, -16.3452) (-24.0666, -16.3471) (-24.0691, -16.349) (-24.0717, -16.351) (-24.0743, -16.353) (-24.077, -16.3551) (-24.0798, -16.3573) (-24.0826, -16.3595) (-24.0855, -16.3618) (-24.0884, -16.3641) (-24.0914, -16.3665) (-24.0945, -16.3689) (-24.0976, -16.3714) (-24.1008, -16.374) (-24.104, -16.3766) (-24.1073, -16.3792) (-24.1107, -16.3819) (-24.1141, -16.3847) (-24.1176, -16.3875) (-24.1211, -16.3904) (-24.1246, -16.3933) (-24.1283, -16.3963) (-24.1319, -16.3994) (-24.1356, -16.4024) (-24.1394, -16.4056) (-24.1432, -16.4088) (-24.1471, -16.412) (-24.151, -16.4153) (-24.155, -16.4187) (-24.159, -16.4221) (-24.1631, -16.4256) (-24.1672, -16.4291) (-24.1713, -16.4326) (-24.1755, -16.4362) (-24.1798, -16.4399) (-24.1841, -16.4436) (-24.1884, -16.4474) (-24.1928, -16.4512) (-24.1972, -16.455) (-24.2017, -16.459) (-24.2062, -16.4629) (-24.2107, -16.4669) (-24.2153, -16.471) (-24.2199, -16.4751) (-24.2246, -16.4793) (-24.2293, -16.4835) (-24.234, -16.4877) (-24.2388, -16.492) (-24.2436, -16.4964) (-24.2485, -16.5008) (-24.2534, -16.5053) (-24.2583, -16.5098) (-24.2633, -16.5143) (-24.2683, -16.5189) (-24.2733, -16.5236) (-24.2784, -16.5282) (-24.2835, -16.533) (-24.2887, -16.5378) (-24.2939, -16.5426) (-24.2991, -16.5475) (-24.3043, -16.5524) (-24.3096, -16.5574) (-24.3149, -16.5624) (-24.3203, -16.5675) (-24.3257, -16.5726) (-24.3311, -16.5778) (-24.3365, -16.583) (-24.342, -16.5882) (-24.3475, -16.5935) (-24.353, -16.5989) (-24.3586, -16.6043) (-24.3642, -16.6097) (-24.3698, -16.6152) (-24.3755, -16.6207) (-24.3812, -16.6263) (-24.3869, -16.6319) (-24.3926, -16.6376) (-24.3984, -16.6433) (-24.4042, -16.6491) (-24.41, -16.6549) (-24.4159, -16.6607) (-24.4218, -16.6666) (-24.4277, -16.6725) (-24.4336, -16.6785) (-24.4395, -16.6845) (-24.4455, -16.6906) (-24.4515, -16.6967) (-24.4576, -16.7029) (-24.4636, -16.7091) (-24.4697, -16.7153) (-24.4758, -16.7216) (-24.482, -16.7279) (-24.4881, -16.7343) (-24.4943, -16.7407) (-24.5005, -16.7472) (-24.5067, -16.7537) (-24.513, -16.7602) (-24.5192, -16.7668) (-24.5255, -16.7735) (-24.5319, -16.7801) (-24.5382, -16.7869) (-24.5446, -16.7936) (-24.5509, -16.8004) (-24.5573, -16.8073) (-24.5638, -16.8142) (-24.5702, -16.8211) (-24.5767, -16.8281) (-24.5831, -16.8351) (-24.5897, -16.8421) (-24.5962, -16.8492) (-24.6027, -16.8564) (-24.6093, -16.8636) (-24.6159, -16.8708) (-24.6225, -16.8781) (-24.6291, -16.8854) (-24.6357, -16.8927) (-24.6424, -16.9001) (-24.6491, -16.9075) (-24.6558, -16.915) (-24.6625, -16.9225) (-24.6692, -16.9301) (-24.6759, -16.9377) (-24.6827, -16.9453) (-24.6895, -16.953) (-24.6963, -16.9607) (-24.7031, -16.9685) (-24.7099, -16.9763) (-24.7168, -16.9841) (-24.7236, -16.992) (-24.7305, -16.9999) (-24.7374, -17.0079) (-24.7443, -17.0159) (-24.7512, -17.0239) (-24.7582, -17.032) (-24.7651, -17.0401) (-24.7721, -17.0483) (-24.7791, -17.0565) (-24.7861, -17.0647) (-24.7931, -17.073) (-24.8001, -17.0813) (-24.8071, -17.0897) (-24.8142, -17.0981) (-24.8212, -17.1065) (-24.8283, -17.115) (-24.8354, -17.1235) (-24.8425, -17.1321) (-24.8496, -17.1407) (-24.8568, -17.1493) (-24.8639, -17.158) (-24.8711, -17.1667) (-24.8782, -17.1754) (-24.8854, -17.1842) (-24.8926, -17.1931) (-24.8998, -17.2019) (-24.907, -17.2108) (-24.9142, -17.2198) (-24.9215, -17.2288) (-24.9287, -17.2378) (-24.936, -17.2469) (-24.9432, -17.2559) (-24.9505, -17.2651) (-24.9578, -17.2743) (-24.9651, -17.2835) (-24.9724, -17.2927) (-24.9797, -17.302) (-24.9871, -17.3113) (-24.9944, -17.3207) (-25.0017, -17.3301) (-25.0091, -17.3395) (-25.0165, -17.349) (-25.0238, -17.3585) (-25.0312, -17.3681) (-25.0386, -17.3777) (-25.046, -17.3873) (-25.0534, -17.397) (-25.0609, -17.4067) (-25.0683, -17.4164) (-25.0757, -17.4262) (-25.0832, -17.436) (-25.0906, -17.4458) (-25.0981, -17.4557) (-25.1055, -17.4657) (-25.113, -17.4756) (-25.1205, -17.4856) (-25.128, -17.4956) (-25.1355, -17.5057) (-25.143, -17.5158) (-25.1505, -17.526) (-25.158, -17.5361) (-25.1655, -17.5464) (-25.1731, -17.5566) (-25.1806, -17.5669) (-25.1881, -17.5772) (-25.1957, -17.5876) (-25.2032, -17.598) (-25.2108, -17.6084) (-25.2184, -17.6189) (-25.2259, -17.6294) (-25.2335, -17.6399) (-25.2411, -17.6505) (-25.2487, -17.6611) (-25.2563, -17.6718) (-25.2639, -17.6825) (-25.2715, -17.6932) (-25.2791, -17.7039) (-25.2867, -17.7147) (-25.2943, -17.7256) (-25.3019, -17.7364) (-25.3096, -17.7473) (-25.3172, -17.7583) (-25.3248, -17.7692) (-25.3325, -17.7802) (-25.3401, -17.7913) (-25.3477, -17.8023) (-25.3539, -17.8112) (-25.3584, -17.8179) (-25.3615, -17.8224) (-25.363, -17.8246) knots 0 0 0 0 0 0 0.00416667 0.00833333 0.0125 0.01666667 0.02083333 0.025 0.02916667 0.03333333 0.0375 0.04166667 0.04583333 0.05 0.05416667 0.05833333 0.0625 0.06666667 0.07083333 0.075 0.07916667 0.08333333 0.0875 0.09166667 0.09583333 0.1 0.10416667 0.10833333 0.1125 0.11666667 0.12083333 0.125 0.12916667 0.13333333 0.1375 0.14166667 0.14583333 0.15 0.15416667 0.15833333 0.1625 0.16666667 0.17083333 0.175 0.17916667 0.18333333 0.1875 0.19166667 0.19583333 0.2 0.20416667 0.20833333 0.2125 0.21666667 0.22083333 0.225 0.22916667 0.23333333 0.2375 0.24166667 0.24583333 0.25 0.25416667 0.25833333 0.2625 0.26666667 0.27083333 0.275 0.27916667 0.28333333 0.2875 0.29166667 0.29583333 0.3 0.30416667 0.30833333 0.3125 0.31666667 0.32083333 0.325 0.32916667 0.33333333 0.3375 0.34166667 0.34583333 0.35 0.35416667 0.35833333 0.3625 0.36666667 0.37083333 0.375 0.37916667 0.38333333 0.3875 0.39166667 0.39583333 0.4 0.40416667 0.40833333 0.4125 0.41666667 0.42083333 0.425 0.42916667 0.43333333 0.4375 0.44166667 0.44583333 0.45 0.45416667 0.45833333 0.4625 0.46666667 0.47083333 0.475 0.47916667 0.48333333 0.4875 0.49166667 0.49583333 0.5 0.50416667 0.50833333 0.5125 0.51666667 0.52083333 0.525 0.52916667 0.53333333 0.5375 0.54166667 0.54583333 0.55 0.55416667 0.55833333 0.5625 0.56666667 0.57083333 0.575 0.57916667 0.58333333 0.5875 0.59166667 0.59583333 0.6 0.60416667 0.60833333 0.6125 0.61666667 0.62083333 0.625 0.62916667 0.63333333 0.6375 0.64166667 0.64583333 0.65 0.65416667 0.65833333 0.6625 0.66666667 0.67083333 0.675 0.67916667 0.68333333 0.6875 0.69166667 0.69583333 0.7 0.70416667 0.70833333 0.7125 0.71666667 0.72083333 0.725 0.72916667 0.73333333 0.7375 0.74166667 0.74583333 0.75 0.75416667 0.75833333 0.7625 0.76666667 0.77083333 0.775 0.77916667 0.78333333 0.7875 0.79166667 0.79583333 0.8 0.80416667 0.80833333 0.8125 0.81666667 0.82083333 0.825 0.82916667 0.83333333 0.8375 0.84166667 0.84583333 0.85 0.85416667 0.85833333 0.8625 0.86666667 0.87083333 0.875 0.87916667 0.88333333 0.8875 0.89166667 0.89583333 0.9 0.90416667 0.90833333 0.9125 0.91666667 0.92083333 0.925 0.92916667 0.93333333 0.9375 0.94166667 0.94583333 0.95 0.95416667 0.95833333 0.9625 0.96666667 0.97083333 0.975 0.97916667 0.98333333 0.9875 0.99166667 0.99583333 1 1 1 1 1 1
  arc A14 (-22.7115, -17.6281) -> (-21.9649, -18.5501) centre (0, 0) ccw
  line L36 (-20.9569, -20.1094) -> (-20.7445, -19.9055)
  line L37 (-27.8937, -8.0945) -> (-27.8945, -8.0948)
  arc A15 (-20.7445, -19.9055) -> (-19.9055, -20.7445) centre (0, 0) ccw
  line L38 (17.8086, -22.9441) -> (17.6281, -22.7115)
  arc A16 (-23.3609, -20.3781) -> (-22.7084, -21.1029) centre (0, 0) ccw
  arc A17 (-30.4202, -5.9675) -> (-30.2174, -6.9214) centre (0, 0) ccw
  arc A18 (-27.918, -6.8665) -> (-27.6109, -8.0125) centre (0, 0) ccw
  spline S17 degree 5 poles (-22.1904, -18.7406) (-22.1905, -18.7407) (-22.1907, -18.7408) (-22.1909, -18.741) (-22.1913, -18.7414) (-22.1919, -18.7419) (-22.1925, -18.7424) (-22.1933, -18.7431) (-22.1941, -18.7438) (-22.195, -18.7446) (-22.196, -18.7455) (-22.197, -18.7464) (-22.1982, -18.7474) (-22.1994, -18.7485) (-22.2007, -18.7497) (-22.202, -18.7509) (-22.2035, -18.7522) (-22.205, -18.7536) (-22.2066, -18.755) (-22.2082, -18.7565) (-22.2099, -18.7581) (-22.2117, -18.7597) (-22.2136, -18.7615) (-22.2155, -18.7632) (-22.2175, -18.7651) (-22.2195, -18.767) (-22.2216, -18.769) (-22.2238, -18.771) (-22.226, -18.7732) (-22.2283, -18.7753) (-22.2307, -18.7776) (-22.2331, -18.7799) (-22.2355, -18.7823) (-22.238, -18.7847) (-22.2406, -18.7872) (-22.2433, -18.7897) (-22.2459, -18.7924) (-22.2487, -18.7951) (-22.2515, -18.7978) (-22.2543, -18.8006) (-22.2572, -18.8035) (-22.2602, -18.8064) (-22.2632, -18.8094) (-22.2662, -18.8124) (-22.2693, -18.8156) (-22.2725, -18.8187) (-22.2757, -18.822) (-22.2789, -18.8252) (-22.2822, -18.8286) (-22.2855, -18.832) (-22.2889, -18.8355) (-22.2923, -18.839) (-22.2958, -18.8426) (-22.2993, -18.8462) (-22.3029, -18.8499) (-22.3065, -18.8536) (-22.3101, -18.8574) (-22.3138, -18.8613) (-22.3175, -18.8652) (-22.3212, -18.8692) (-22.325, -18.8732) (-22.3289, -18.8773) (-22.3328, -18.8814) (-22.3367, -18.8856) (-22.3406, -18.8899) (-22.3446, -18.8942) (-22.3486, -18.8986) (-22.3527, -18.903) (-22.3568, -18.9074) (-22.3609, -18.9119) (-22.3651, -18.9165) (-22.3693, -18.9211) (-22.3736, -18.9258) (-22.3778, -18.9306) (-22.3821, -18.9353) (-22.3865, -18.9402) (-22.3909, -18.9451) (-22.3953, -18.95) (-22.3997, -18.955) (-22.4042, -18.96) (-22.4087, -18.9651) (-22.4132, -18.9703) (-22.4177, -18.9755) (-22.4223, -18.9807) (-22.427, -18.986) (-22.4316, -18.9914) (-22.4363, -18.9968) (-22.441, -19.0022) (-22.4457, -19.0077) (-22.4505, -19.0133) (-22.4553, -19.0189) (-22.4601, -19.0246) (-22.4649, -19.0303) (-22.4698, -19.036) (-22.4747, -19.0418) (-22.4796, -19.0477) (-22.4846, -19.0536) (-22.4895, -19.0595) (-22.4945, -19.0655) (-22.4996, -19.0715) (-22.5046, -19.0776) (-22.5097, -19.0838) (-22.5148, -19.09) (-22.5199, -19.0962) (-22.525, -19.1025) (-22.5302, -19.1088) (-22.5354, -19.1152) (-22.5406, -19.1216) (-22.5458, -19.1281) (-22.5511, -19.1346) (-22.5564, -19.1412) (-22.5617, -19.1478) (-22.567, -19.1544) (-22.5723, -19.1611) (-22.5777, -19.1679) (-22.583, -19.1747) (-22.5884, -19.1815) (-22.5939, -19.1884) (-22.5993, -19.1954) (-22.6048, -19.2024) (-22.6102, -19.2094) (-22.6157, -19.2165) (-22.6212, -19.2236) (-22.6268, -19.2307) (-22.6323, -19.2379) (-22.6379, -19.2452) (-22.6435, -19.2525) (-22.6491, -19.2598) (-22.6547, -19.2672) (-22.6603, -19.2747) (-22.666, -19.2821) (-22.6716, -19.2897) (-22.6773, -19.2972) (-22.683, -19.3048) (-22.6887, -19.3125) (-22.6945, -19.3202) (-22.7002, -19.3279) (-22.706, -19.3357) (-22.7118, -19.3436) (-22.7175, -19.3514) (-22.7233, -19.3593) (-22.7292, -19.3673) (-22.735, -19.3753) (-22.7408, -19.3834) (-22.7467, -19.3914) (-22.7526, -19.3996) (-22.7585, -19.4078) (-22.7644, -19.416) (-22.7703, -19.4242) (-22.7762, -19.4325) (-22.7822, -19.4409) (-22.7881, -19.4493) (-22.7941, -19.4577) (-22.8, -19.4662) (-22.806, -19.4747) (-22.812, -19.4832) (-22.818, -19.4918) (-22.8241, -19.5005) (-22.8301, -19.5091) (-22.8361, -19.5179) (-22.8422, -19.5266) (-22.8483, -19.5354) (-22.8543, -19.5443) (-22.8604, -19.5532) (-22.8665, -19.5621) (-22.8726, -19.5711) (-22.8787, -19.5801) (-22.8849, -19.5891) (-22.891, -19.5982) (-22.8971, -19.6073) (-22.9033, -19.6165) (-22.9095, -19.6257) (-22.9156, -19.635) (-22.9218, -19.6443) (-22.928, -19.6536) (-22.9342, -19.663) (-22.9404, -19.6724) (-22.9466, -19.6818) (-22.9528, -19.6913) (-22.9591, -19.7009) (-22.9653, -19.7104) (-22.9715, -19.72) (-22.9778, -19.7297) (-22.984, -19.7394) (-22.9903, -19.7491) (-22.9966, -19.7589) (-23.0029, -19.7687) (-23.0091, -19.7785) (-23.0154, -19.7884) (-23.0217, -19.7984) (-23.028, -19.8083) (-23.0343, -19.8183) (-23.0406, -19.8284) (-23.047, -19.8384) (-23.0533, -19.8486) (-23.0596, -19.8587) (-23.066, -19.8689) (-23.0723, -19.8791) (-23.0786, -19.8894) (-23.085, -19.8997) (-23.0914, -19.9101) (-23.0977, -19.9205) (-23.1041, -19.9309) (-23.1104, -19.9413) (-23.1168, -19.9518) (-23.1232, -19.9624) (-23.1296, -19.973) (-23.136, -19.9836) (-23.1423, -19.9942) (-23.1487, -20.0049) (-23.1551, -20.0156) (-23.1615, -20.0264) (-23.1679, -20.0372) (-23.1743, -20.048) (-23.1807, -20.0589) (-23.1872, -20.0698) (-23.1936, -20.0808) (-23.2, -20.0917) (-23.2064, -20.1028) (-23.2128, -20.1138) (-23.2193, -20.1249) (-23.2257, -20.136) (-23.2321, -20.1472) (-23.2385, -20.1584) (-23.245, -20.1697) (-23.2514, -20.1809) (-23.2578, -20.1922) (-23.2643, -20.2036) (-23.2707, -20.215) (-23.2771, -20.2264) (-23.2836, -20.2379) (-23.29, -20.2493) (-23.2965, -20.2609) (-23.3029, -20.2724) (-23.3094, -20.284) (-23.3158, -20.2957) (-23.3222, -20.3073) (-23.3287, -20.319) (-23.3351, -20.3308) (-23.3416, -20.3426) (-23.348, -20.3544) (-23.3532, -20.3639) (-23.3571, -20.371) (-23.3596, -20.3757) (-23.3609, -20.3781) knots 0 0 0 0 0 0 0.00416667 0.00833333 0.0125 0.01666667 0.02083333 0.025 0.02916667 0.03333333 0.0375 0.04166667 0.04583333 0.05 0.05416667 0.05833333 0.0625 0.06666667 0.07083333 0.075 0.07916667 0.08333333 0.0875 0.09166667 0.09583333 0.1 0.10416667 0.10833333 0.1125 0.11666667 0.12083333 0.125 0.12916667 0.13333333 0.1375 0.14166667 0.14583333 0.15 0.15416667 0.15833333 0.1625 0.16666667 0.17083333 0.175 0.17916667 0.18333333 0.1875 0.19166667 0.19583333 0.2 0.20416667 0.20833333 0.2125 0.21666667 0.22083333 0.225 0.22916667 0.23333333 0.2375 0.24166667 0.24583333 0.25 0.25416667 0.25833333 0.2625 0.26666667 0.27083333 0.275 0.27916667 0.28333333 0.2875 0.29166667 0.29583333 0.3 0.30416667 0.30833333 0.3125 0.31666667 0.32083333 0.325 0.32916667 0.33333333 0.3375 0.34166667 0.34583333 0.35 0.35416667 0.35833333 0.3625 0.36666667 0.37083333 0.375 0.37916667 0.38333333 0.3875 0.39166667 0.39583333 0.4 0.40416667 0.40833333 0.4125 0.41666667 0.42083333 0.425 0.42916667 0.43333333 0.4375 0.44166667 0.44583333 0.45 0.45416667 0.45833333 0.4625 0.46666667 0.47083333 0.475 0.47916667 0.48333333 0.4875 0.49166667 0.49583333 0.5 0.50416667 0.50833333 0.5125 0.51666667 0.52083333 0.525 0.52916667 0.53333333 0.5375 0.54166667 0.54583333 0.55 0.55416667 0.55833333 0.5625 0.56666667 0.57083333 0.575 0.57916667 0.58333333 0.5875 0.59166667 0.59583333 0.6 0.60416667 0.60833333 0.6125 0.61666667 0.62083333 0.625 0.62916667 0.63333333 0.6375 0.64166667 0.64583333 0.65 0.65416667 0.65833333 0.6625 0.66666667 0.67083333 0.675 0.67916667 0.68333333 0.6875 0.69166667 0.69583333 0.7 0.70416667 0.70833333 0.7125 0.71666667 0.72083333 0.725 0.72916667 0.73333333 0.7375 0.74166667 0.74583333 0.75 0.75416667 0.75833333 0.7625 0.76666667 0.77083333 0.775 0.77916667 0.78333333 0.7875 0.79166667 0.79583333 0.8 0.80416667 0.80833333 0.8125 0.81666667 0.82083333 0.825 0.82916667 0.83333333 0.8375 0.84166667 0.84583333 0.85 0.85416667 0.85833333 0.8625 0.86666667 0.87083333 0.875 0.87916667 0.88333333 0.8875 0.89166667 0.89583333 0.9 0.90416667 0.90833333 0.9125 0.91666667 0.92083333 0.925 0.92916667 0.93333333 0.9375 0.94166667 0.94583333 0.95 0.95416667 0.95833333 0.9625 0.96666667 0.97083333 0.975 0.97916667 0.98333333 0.9875 0.99166667 0.99583333 1 1 1 1 1 1
  line L39 (22.7115, -17.6281) -> (22.9441, -17.8086)